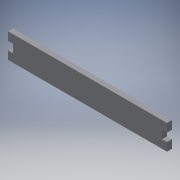
# Autodesk Inventor part: Деталь7
Saved by Autodesk Inventor 2019 (Build 230136000, 136)
## iProperties
Created: 2022-02-24
Part Number: Деталь7
Material: Типовые
Document SubType Name: Modeling
Designer: korsh
Density: 1 g/cm^3
Appearance: По умолчанию
Author: korsh
Autodesk Inventor part; units mm, degrees
ref_plane "YZ Plane" through (0, 0, 0) normal (1, 0, 0) x (0, 1, 0)
ref_plane "XZ Plane" through (0, 0, 0) normal (0, 1, 0) x (-1, 0, 0)
ref_plane "XY Plane" through (0, 0, 0) normal (0, 0, 1) x (1, 0, 0)
sketch "Эскиз1" plane through (0, 0, 0) normal (0, 0, 1) x (1, 0, 0)
  line L0 (0, 0) -> (180, 0)
  line L1 (180, 0) -> (180, -30)
  line L2 (180, -30) -> (0, -30)
  line L3 (0, -30) -> (0, 0)
  line L4 (0, 0) -> (-6, 0)
  line L5 (-6, 0) -> (-6, -10)
  line L6 (-6, -10) -> (0, -10)
  line L7 (0, -10) -> (0, 0)
  line L8 (0, -20) -> (-6, -20)
  line L9 (-6, -20) -> (-6, -30)
  line L10 (-6, -30) -> (0, -30)
  line L11 (0, -30) -> (0, -20)
  line L12 (180, 0) -> (186, 0)
  line L13 (186, 0) -> (186, -10)
  line L14 (186, -10) -> (180, -10)
  line L15 (180, -10) -> (180, 0)
  line L16 (180, -30) -> (180, -20)
  line L17 (186, -20) -> (186, -30)
  line L18 (186, -30) -> (180, -30)
  line L19 (180, -20) -> (186, -20)
  dimension "d0" = 180
  dimension "d1" = 30
  dimension "d2" = 10
  dimension "d3" = 6
  dimension "d6" = 20
  dimension "d11" = 6
  dimension "d14" = 20
  constraints: 40 end point, 6 parallel, 3 horizontal, 3 perpendicular, 2 vertical, 16 other
  measures "d0" distance of L1.end L2.end
  measures "d1" distance of L0.end L1.end
  measures "d2" distance of L4.end L5.end
  measures "d3" distance of L5.end L6.end
  measures "d6" distance of L5.end L9.end
  measures "d11" distance of L13.end L14.end
  measures "d14" distance of L0.end L16.end
extrude "Выдавливание1" add sketch "Эскиз1" along normal blind 6
